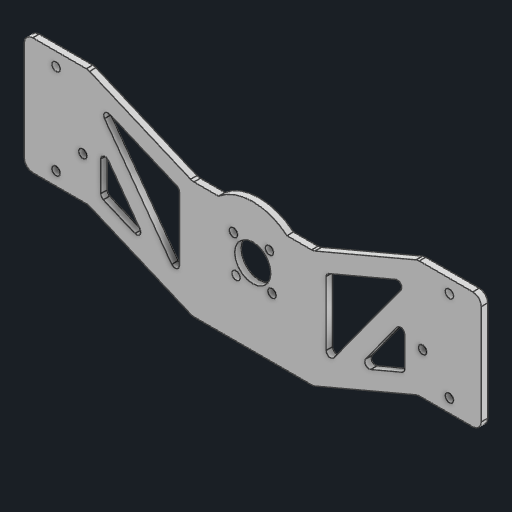
# Autodesk Inventor part: NeckBase
Saved by Autodesk Inventor 2025.2 (Build 292293000, 293)
## iProperties
Created: 2025-08-15
Part Number: NeckBase
Material: Generic
Document SubType Name: Sheet Metal
Designer: valer
Density: 1 g/cm^3
Sheet Metal Rule: Default
Appearance: Default
Author: valer
Autodesk Inventor part; units mm, degrees
ref_plane "YZ Plane" through (0, 0, 0) normal (1, 0, 0) x (0, 1, 0)
ref_plane "XZ Plane" through (0, 0, 0) normal (0, 1, 0) x (-1, 0, 0)
ref_plane "XY Plane" through (0, 0, 0) normal (0, 0, 1) x (1, 0, 0)
sketch "Sketch1" plane through (0, 0, 0) normal (0, 0, 1) x (1, 0, 0)
  circle A0 centre (0, 7.375) radius 19.125 construction
  line L0 (0, -28.5) -> (-28.5, -28.5)
  line L1 (-28.5, -28.5) -> (-77.549, -7.6799)
  line L2 (-77.549, 47.3201) -> (-28.5, 26.5)
  line L3 (-28.5, 26.5) -> (0, 26.5)
  line L4 (0, -43.664) -> (0, 62.4841) construction
  line L5 (-28.5, -28.5) -> (-28.5, 26.5) construction
  line L6 (-77.549, -7.6799) -> (-77.549, 47.3201) construction
  circle A1 centre (0, 7.375) radius 25
  line L7 (28.5, -28.5) -> (77.549, -7.6799)
  line L8 (107.549, -7.6799) -> (77.549, 47.3201) construction
  line L9 (77.549, 47.3201) -> (28.5, 26.5)
  line L10 (28.5, 26.5) -> (0, 26.5)
  line L11 (-28.5, 24.5) -> (-28.5, -24.5) construction
  line L12 (-34.5, 20.356) -> (-34.5, -17.2623)
  line L13 (-34.5, -17.2623) -> (-74.0188, 37.1307)
  line L14 (-48.798, -11.1931) -> (-71.549, 20.1209)
  line L15 (-71.549, 20.1209) -> (-71.549, -1.5359)
  line L16 (-71.549, -1.5359) -> (-48.798, -11.1931)
  line L17 (-34.5, -17.2623) -> (-48.798, -11.1931) construction
  line L18 (-34.5, 20.356) -> (-74.0188, 37.1307)
  line L19 (34.5, 20.356) -> (34.5, -17.2623)
  line L20 (34.5, -17.2623) -> (74.0188, 37.1307)
  line L21 (48.798, -11.1931) -> (71.549, 20.1209)
  line L22 (71.549, 20.1209) -> (71.549, -1.5359)
  line L23 (71.549, -1.5359) -> (48.798, -11.1931)
  line L24 (34.5, 20.356) -> (74.0188, 37.1307)
  line L25 (28.5, -28.5) -> (0, -28.5)
  line L26 (-74.0188, 37.1307) -> (-71.549, 20.1209) construction
  line L27 (107.549, -7.6799) -> (107.549, 47.3201)
  line L28 (77.549, 47.3201) -> (107.549, 47.3201)
  line L29 (107.549, -7.6799) -> (77.549, -7.6799)
  line L30 (77.549, -7.6799) -> (77.549, 47.3201) construction
  line L31 (-107.549, -7.6799) -> (-77.549, 47.3201) construction
  line L32 (-107.549, -7.6799) -> (-107.549, 47.3201)
  line L33 (-77.549, 47.3201) -> (-107.549, 47.3201)
  line L34 (-107.549, -7.6799) -> (-77.549, -7.6799)
  point P0 (0, 0)
  point P1 (-77.549, 19.8201)
  point P2 (16.1008, 26.5)
  point P3 (-16.1008, 26.5)
  dimension "d1" = 50
  dimension "d6" = 6
  dimension "d7" = 6
  dimension "d8" = 8
  dimension "d9" = 8
  dimension "d10" = 8
  dimension "d11" = 36
  dimension "d29" = 157
  dimension "d30" = 157
  dimension "d32" = 157
  dimension "d33" = 49.049
  dimension "d34" = 28.5
  dimension "d38" = 28.5
  dimension "d39" = 5.875
  dimension "d41" = 37.6182
  dimension "d42" = 8
  dimension "d43" = 6
  dimension "d45" = 55
  dimension "d46" = 30
  measures "d1" diameter of A1
  measures "d6" distance between parallel lines of L11 L12
  measures "d7" distance from line of point (-77.549, 19.82) L15
  measures "d8" distance between parallel lines of L1 L16
  measures "d9" distance between parallel lines of L2 L18
  measures "d10" distance between parallel lines of L14 L13
  measures "d11" angle of L12 L13
  measures "d29" angle of L25 L7
  measures "d30" angle of L1 L0
  measures "d32" angle of L2 L3
  measures "d33" horizontal distance of L7.start L7.end
  measures "d34" distance of L7.start L0.start
  measures "d38" distance from line of L25 point (0, 0)
  measures "d39" radial gap between concentric circles of A0 A1
  measures "d41" distance of L19.start L19.end
  measures "d42" distance between parallel lines of L20 L21
  measures "d43" distance from line of L7.end L22
  measures "d45" distance of L8.start L27.end
  measures "d46" distance of L8.start L7.end
extrude "Plate1" add sketch "Sketch1" along normal blind 3.048
fillet "OutsideFilletsFeature" radius 4 12 edges at (107.549, -7.6799, 1.524) (-28.5, -28.5, 1.524) (28.5, -28.5, 1.524) (-28.5, 26.5, 1.524) (28.5, 26.5, 1.524) (77.549, 47.3201, 1.524) (-77.549, 47.3201, 1.524) (-107.549, -7.6799, 1.524) (-77.549, -7.6799, 1.524) (77.549, -7.6799, 1.524) (107.549, 47.3201, 1.524) (-107.549, 47.3201, 1.524)
fillet "InsideFilletsFeature" radius 2 12 edges at (71.549, -1.5359, 1.524) (48.798, -11.1931, 1.524) (34.5, 20.356, 1.524) (34.5, -17.2623, 1.524) (74.0188, 37.1307, 1.524) (-34.5, -17.2623, 1.524) (-34.5, 20.356, 1.524) (-74.0188, 37.1307, 1.524) (-48.798, -11.1931, 1.524) (-71.549, -1.5359, 1.524) (-71.549, 20.1209, 1.524) (71.549, 20.1209, 1.524)
sketch "BracketMountHoles" plane through (0, 0, 3.048) normal (0, 0, 1) x (1, 0, 0)
  circle A0 centre (92.549, -1.4166) radius 2 projected
  circle A1 centre (92.549, 41.0567) radius 2 projected
  point P0 (0, 0)
hole "BracketMountHolesFeature" at (92.549, -1.4166, 3.048) at (92.549, 41.0567, 3.048) direction (0, 0, -1) diameter 4 depth 3.048 tip angle 118
mirror "BracketMountHolesMirrorFeature" about plane through (0, 0, 0) normal (1, 0, 0) of "BracketMountHolesFeature"
sketch "FlangeMountHoles" plane through (0, 0, 3.048) normal (0, 0, 1) x (1, 0, 0)
  circle A0 centre (-9.0729, 15.2288) radius 2 projected
  circle A1 centre (7.8538, 16.4479) radius 2 projected
  circle A2 centre (9.0729, -0.4788) radius 2 projected
  circle A3 centre (-7.8538, -1.6979) radius 2 projected
  point P0 (0, 0)
extrude "FlangeMountHolesFeature" cut sketch "FlangeMountHoles" against normal blind 3.048
sketch "ActuatorMountHoles" plane through (0, 0, 3.048) normal (0, 0, 1) x (1, 0, 0)
  circle A0 centre (79.9496, 11.9377) radius 2 projected
  circle A1 centre (-79.9496, 11.9377) radius 2 projected
  point P0 (0, 0)
extrude "ActuatorMountHolesFeature" cut sketch "ActuatorMountHoles" against normal blind 3.048
sketch "FlangeCut" plane through (0, 0, 3.048) normal (0, 0, 1) x (1, 0, 0)
  circle A0 centre (0, 7.375) radius 8 construction
  circle A1 centre (0, 7.375) radius 8.5
  point P0 (0, 0)
  dimension "d65" = 0.5
  constraints: 1 centre point, 1 coincident
  measures "d65" radial gap between concentric circles of A1 A0
extrude "FlangeCutFeature" cut sketch "FlangeCut" against normal blind 3.048
equation "\"d12\" = Thickness"
equation "\"BendRadius\" = Thickness"
equation "\"BendReliefWidth\" = Thickness"
equation "\"BendReliefDepth\" = 0.5 * Thickness"
equation "\"CornerReliefSize\" = 4 * Thickness"
equation "\"MinimumRemnant\" = 2 * Thickness"
equation "\"TransitionRadius\" = BendRadius"
equation "\"JacobiRadiusSize\" = BendRadius"
equation "\"GapSize\" = Thickness"
equation "\"Thickness\" = 3.048"
body "Solid1"
